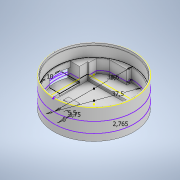
# Autodesk Inventor part: t2
Saved by Autodesk Inventor 2022.2 (Build 262287000, 287)
## iProperties
Created: 2022-04-08
Part Number: t2
Material: Generic
Document SubType Name: Modeling
Designer: 21towe
Density: 1 g/cm^3
Appearance: Default
Author: 21towe
Autodesk Inventor part; units mm, degrees
ref_plane "YZ Plane" through (0, 0, 0) normal (1, 0, 0) x (0, 1, 0)
ref_plane "XZ Plane" through (0, 0, 0) normal (0, 1, 0) x (-1, 0, 0)
ref_plane "XY Plane" through (0, 0, 0) normal (0, 0, 1) x (1, 0, 0)
sketch "Sketch1" plane through (0, 0, 0) normal (0, 1, 0) x (-1, 0, 0)
  circle A0 centre (0, 0) radius 20
  dimension "d0" = 40
  constraints: 1 centre point, 1 coincident
  measures "d0" diameter of A0
extrude "Extrusion1" add sketch "Sketch1" along normal blind 0.5
sketch "Sketch2" plane through (0, 0.5, 0) normal (0, 1, 0) x (1, 0, 0)
  line L0 (-13.25, -10) -> (13.25, -10)
  line L1 (13.25, -10) -> (13.25, 10)
  line L2 (13.25, 10) -> (-13.25, 10)
  line L3 (-13.25, 10) -> (-13.25, -10)
  line L4 (-13.25, -10) -> (13.25, 10) construction
  line L5 (13.25, -10) -> (-13.25, 10) construction
  circle A0 centre (0, 0) radius 20
  dimension "d3" = 26.5
  dimension "d4" = 20
  constraints: 12 end point, 2 midpoint, 2 parallel, 1 centre point, 1 coincident, 1 horizontal, 1 perpendicular
  measures "d3" distance of L2.end L1.end
  measures "d4" distance of L1.end L0.end
extrude "Extrusion2" add sketch "Sketch2" along normal blind 3
ref_plane "Work Plane1" through (0, 3.5, 0) normal (0, 1, 0) x (1, 0, 0)
sketch "Sketch3" plane through (0, 3.5, 0) normal (0, 1, 0) x (1, 0, 0)
  line L0 (16.25, 0) -> (16.25, 3)
  line L1 (16.25, 3) -> (18.2551, 3)
  line L2 (16.25, 0) -> (16.25, -3)
  line L3 (16.25, -3) -> (18.2551, -3)
  line L4 (0, -18.5) -> (0, -12.5)
  line L5 (0, -12.5) -> (2.75, -12.5)
  line L6 (2.75, -12.5) -> (-2.75, -12.5)
  line L7 (-2.75, -12.5) -> (-2.75, -10)
  line L8 (-2.75, -10) -> (2.75, -10)
  line L9 (2.75, -10) -> (2.75, -12.5)
  line L10 (-17.5, 6) -> (-13.25, 6)
  line L11 (-12.5, 10) -> (-12.5, 13.6382)
  line L12 (0, 18.5) -> (0, 16.5)
  line L13 (0, 16.5) -> (-8.3666, 16.5)
  line L14 (18.2551, -3) -> (15.4901, -3)
  line L15 (15.4901, -3) -> (15.4901, 3)
  line L16 (15.4901, 3) -> (16.25, 3)
  circle A0 centre (0, 0) radius 18.75
  line L17 (18.2551, 3) -> (18.5084, 3)
  line L18 (18.2551, -3) -> (18.5084, -3)
  line L19 (0, 18.5) -> (0, 18.75)
  line L20 (-8.3666, 16.5) -> (-8.9058, 16.5)
  line L21 (-17.5, 6) -> (-17.7641, 6)
  line L22 (-12.5, 13.6382) -> (-12.5, 13.9754)
  line L23 (-13.25, 10) -> (13.25, 10) projected
  line L24 (-12.5, 10) -> (-13.25, 10)
  line L25 (-13.25, 10) -> (-13.25, 6)
  line L26 (-13.25, -10) -> (-13.25, 10) projected
  circle A1 centre (0, 0) radius 20
  dimension "d8" = 6
  dimension "d9" = 2.75
  dimension "d10" = 5.5
  dimension "d11" = 2
  dimension "d12" = 2.765
  dimension "d13" = 37.5
  constraints: 50 end point, 9 perpendicular, 7 point on line, 6 point on circle, 2 centre point, 2 coincident, 1 collinear, 1 parallel, 2 other
  measures "d8" distance of L4.start L4.end
  measures "d9" distance of L4.end L5.end
  measures "d10" distance of L5.end L6.end
  measures "d11" distance of L12.start L12.end
  measures "d12" distance of L3.end L14.end
  measures "d13" diameter of A0
extrude "Extrusion3" cut sketch "Sketch3" against normal blind 1.5 contours L16 L15 L14 L3 L18 A0 L21 L10 L25 L23 L11 L22 L20 L13 L12 L19 L17 L1
extrude "Extrusion4" add sketch "Sketch3" along normal blind 5.25 contours L2 L14 L15 L16 L0 | L0 L1 L17 A0 L18 L3 L2 | L19 L12 L13 L20 A0 | A0 L22 L11 L23 L25 L10 L21 | L6 L7 L8 L9 L5
extrude "Extrusion5" add sketch "Sketch3" along normal blind 5.25 contours A1
sketch "Sketch4" plane through (0, 2, 0) normal (0, 1, 0) x (1, 0, 0)
  line L0 (14.25, -9) -> (12.25, -9)
  line L1 (12.25, -9) -> (12.25, -11)
  line L2 (12.25, -11) -> (14.25, -11)
  line L3 (14.25, -11) -> (14.25, -9)
  line L4 (2.75, -10) -> (13.25, -10) projected
  line L5 (14.25, -9) -> (12.25, -11) construction
  line L6 (12.25, -9) -> (14.25, -11) construction
  point P0 (0, 0)
  dimension "d20" = 2
  dimension "d21" = 2
  constraints: 12 end point, 2 midpoint, 2 parallel, 1 horizontal, 1 perpendicular
  measures "d20" distance of L2.end L1.end
  measures "d21" distance of L1.end L0.end
extrude "Extrusion6" cut sketch "Sketch4" against normal blind 1.5
sketch "Sketch5" plane through (0, 8.75, 0) normal (0, 1, 0) x (1, 0, 0)
  circle A0 centre (0, 0) radius 19.25
  circle A1 centre (0, 0) radius 20
  circle A2 centre (0, 0) radius 19.5
  dimension "d24" = 38.5
  dimension "d25" = 39
  constraints: 3 centre point, 3 coincident
  measures "d24" diameter of A0
  measures "d25" diameter of A2
extrude "Extrusion7" add sketch "Sketch5" along normal blind 5 contours A1 | A2
extrude "Extrusion8" add sketch "Sketch5" along normal blind 6 contours A1
sketch "Sketch6" plane through (0, 14.75, 0) normal (0, 1, 0) x (1, 0, 0)
  line L0 (-0.2579, -20.6923) -> (0.2579, -20.6923)
  line L1 (0.2579, -20.6923) -> (0.2579, -19.3077)
  line L2 (0.2579, -19.3077) -> (-0.2579, -19.3077)
  line L3 (-0.2579, -19.3077) -> (-0.2579, -20.6923)
  circle A0 centre (0, 0) radius 20 projected
  line L4 (-0.2579, -20.6923) -> (0.2579, -19.3077) construction
  line L5 (0.2579, -20.6923) -> (-0.2579, -19.3077) construction
  point P0 (0, -20)
  constraints: 12 end point, 2 midpoint, 2 parallel, 1 horizontal, 1 perpendicular, 1 vertical alignment, 1 other
extrude "Extrusion9" add sketch "Sketch6" along normal blind 1 contours L3 A0 L1 L0 | L3 L2 L1 A0 picked at (-0.0287, -19.5384)
sketch "Sketch7" plane through (0.2579, 14.75, 20.6923) normal (1, 0, 0) x (0, 0, -1)
  line L0 (0, 0) -> (0.6939, 0) projected
  line L1 (0.6939, 0) -> (0.9439, 0)
  line L2 (1.194, 0) -> (0.6939, 0) projected
  circle A0 centre (0.9439, 0) radius 0.25
  line L3 (1.194, 0) -> (1.3845, 0) projected
  line L4 (1.194, 0) -> (2.041, 0)
  point P0 (20.6923, -14.75)
  point P1 (0.6939, 0)
  dimension "d32" = 0.25
  constraints: 4 end point, 1 coincident, 1 horizontal, 1 point on line, 3 other
  measures "d32" distance of L0.end L1.end
extrude "Extrusion10" cut sketch "Sketch6" along normal blind 1 contours L3 A0 L1 L0 | L3 L2 L1 A0 picked at (-0.0287, -19.5384)
sketch3d "3D Sketch1"
  arc A0 (0.2579, 14.75, 19.4983) -> (-19.4983, 14.75, 0.2579) centre (0, 14.75, 0) ccw
  arc A1 (-19.4983, 14.75, 0.2579) -> (-0.2579, 14.75, -19.4983) centre (0, 14.75, 0) ccw
  arc A2 (-0.2579, 14.75, -19.4983) -> (19.4983, 14.75, -0.2579) centre (0, 14.75, 0) ccw
  arc A3 (19.4983, 14.75, -0.2579) -> (0.2579, 14.75, 19.4983) centre (0, 14.75, 0) ccw
sweep "Sweep1" add profiles "Sketch7" path "3D Sketch1" picked at (1.1082, 0.0199) contours A0 L2 L1
sketch "Sketch8" plane through (0, 2, 0) normal (0, 1, 0) x (1, 0, 0)
  line L0 (-17.7641, 6) -> (-13.25, 6) projected
  line L1 (-13.25, 6) -> (-22.0504, 6)
  line L2 (-22.0504, 6) -> (-22.0504, -4)
  line L3 (-22.0504, -4) -> (-13.25, -4)
  line L4 (-13.25, -4) -> (-13.25, 6)
  point P0 (0, 0)
  dimension "d37" = 10
  constraints: 8 end point, 2 parallel, 1 horizontal, 1 perpendicular
  measures "d37" distance of L2.end L1.end
extrude "Extrusion11" cut sketch "Sketch8" against normal blind 1
extrude "Extrusion12" cut sketch "Sketch8" along normal blind 3
extrude "Extrusion13" cut sketch "Sketch8" along normal blind 4
body "Solid1"
